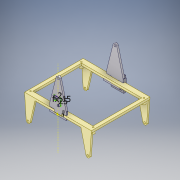
# Autodesk Inventor part: ControllerPCBHolder
Saved by Autodesk Inventor 2019.1 (Build 231200000, 200)
## iProperties
Created: 2018-09-15
Part Number: ControllerPCBHolder
Material: Generisch
Document SubType Name: Modeling
Designer: JochenAlt
Density: 1 g/cm^3
Appearance: Nylon 6
Author: JochenAlt
Autodesk Inventor part; units mm, degrees
ref_plane "YZ Plane" through (0, 0, 0) normal (1, 0, 0) x (0, 1, 0)
ref_plane "XZ Plane" through (0, 0, 0) normal (0, 1, 0) x (-1, 0, 0)
ref_plane "XY Plane" through (0, 0, 0) normal (0, 0, 1) x (1, 0, 0)
sketch "Skizze1" plane through (0, 0, 0) normal (0, 0, 1) x (1, 0, 0)
  line L0 (-61, 50.5) -> (61, 50.5)
  line L1 (61, 50.5) -> (61, -50.5)
  line L2 (61, -50.5) -> (-61, -50.5)
  line L3 (-61, -50.5) -> (-61, 50.5)
  line L4 (0, 70.7) -> (0, -70.7) construction
  line L5 (-85.4, 0) -> (85.4, 0) construction
  line L6 (-55, 44.5) -> (55, 44.5)
  line L7 (55, 44.5) -> (55, -44.5)
  line L8 (55, -44.5) -> (-55, -44.5)
  line L9 (-55, -44.5) -> (-55, 44.5)
  line L10 (-57.15, 46.36) -> (57.15, 46.36) construction
  line L11 (57.15, 46.36) -> (57.15, -46.36) construction
  line L12 (57.15, -46.36) -> (-57.15, -46.36) construction
  line L13 (-57.15, -46.36) -> (-57.15, 46.36) construction
  circle A0 centre (-57.15, 46.36) radius 1.25
  circle A1 centre (57.15, 46.36) radius 1.25
  circle A2 centre (-57.15, -46.36) radius 1.25
  circle A3 centre (57.15, -46.36) radius 1.25
  circle A4 centre (57.15, 46.36) radius 2.8429
  circle A5 centre (-57.15, 46.36) radius 2.8429
  circle A6 centre (-57.15, -46.36) radius 2.8429
  circle A7 centre (57.15, -46.36) radius 2.8429
  point P0 (0, 0)
  dimension "d0" = 122
  dimension "d1" = 101
  dimension "d4" = 6
  dimension "d5" = 6
  dimension "d6" = 2.5
  dimension "d7" = 114.3
  dimension "d8" = 92.72
  constraints: 24 end point, 8 coincident, 6 parallel, 4 centre point, 3 equal radius, 3 horizontal, 3 perpendicular, 18 other
  measures "d0" distance of L0.start L0.end
  measures "d1" distance of L0.end L1.end
  measures "d4" distance between parallel lines of L6 L0
  measures "d5" distance between parallel lines of L9 L3
  measures "d6" diameter of A0
  measures "d7" distance of L11.end L12.end
  measures "d8" distance of L10.end L11.end
extrude "Extrusion2" add sketch "Skizze1" along normal blind 4 contours L0 L1 L2 L3 | A4 | A7 | A6 | A5
extrude "Extrusion15" add sketch "Skizze1" against normal blind 5 contours A4 | A7 | A6 | A5
sketch "Skizze2" plane through (0, 0, 0) normal (0, 1, 0) x (-1, 0, 0)
  arc A0 (51.152, -39.299) -> (58.0513, -38.7409) centre (54.5596, -38.5) ccw
  arc A1 (-58.0513, -38.7409) -> (-51.152, -39.299) centre (-54.5596, -38.5) ccw
  line L0 (0, -100.1) -> (0, 86.1) construction
  line L1 (-93.1, 0) -> (93.1, 0) construction
  circle A2 centre (54.5596, -38.5) radius 1.75
  circle A3 centre (-54.5596, -38.5) radius 1.75
  line L2 (58.0513, -38.7409) -> (61, 4)
  line L3 (-58.0513, -38.7409) -> (-61, 4)
  line L4 (-61, 4) -> (61, 4) construction
  line L5 (61, 4) -> (41, 4)
  line L6 (-61, 4) -> (-41, 4)
  circle A4 centre (0, 56) radius 1.75
  arc A5 (3.3952, 56.8501) -> (-3.3952, 56.8501) centre (0, 56) ccw
  line L7 (54.5596, -38.5) -> (0, 56) construction
  line L8 (61, 0) -> (-61, 0) construction
  circle A6 centre (0, -7) radius 63 construction
  line L9 (54.5596, -38.5) -> (-54.5596, -38.5) construction
  line L10 (0, 56) -> (-54.5596, -38.5) construction
  line L11 (55, 4) -> (-55, 4) construction
  line L12 (7, 0) -> (7, 0)
  line L13 (7, 0) -> (-7, 0)
  line L14 (7, 4.5) -> (15, 4.5)
  line L15 (15, 4.5) -> (15, 10.0685)
  line L16 (-15, 10.0685) -> (-15, 4.5)
  line L17 (-15, 4.5) -> (-7, 4.5)
  line L18 (7, 9.5) -> (-7, 9.5)
  line L19 (7, 9.5) -> (7, 0)
  line L20 (-7, 9.5) -> (-7, 0)
  line L21 (-3.3952, 56.8501) -> (-14.8952, 10.9186)
  line L22 (3.3952, 56.8501) -> (14.8952, 10.9186)
  arc A7 (-14.8952, 10.9186) -> (-15, 10.0685) centre (-11.5, 10.0685) ccw
  arc A8 (15, 10.0685) -> (14.8952, 10.9186) centre (11.5, 10.0685) ccw
  line L23 (-51.152, -39.299) -> (-41, 4)
  line L24 (51.152, -39.299) -> (41, 4)
  line L25 (-61, 0) -> (-61, 4) projected
  circle A9 centre (0, -7) radius 66.5 construction
  point P0 (0, 0)
  point P1 (15, 10.5)
  dimension "d12" = 3.5
  dimension "d22" = 63
  dimension "d23" = 3.5
  dimension "d54" = 6
  dimension "d61" = 30
  dimension "d71" = 0.5
  dimension "d74" = 7
  dimension "d76" = 5
  dimension "d81" = 20
  dimension "d82" = 14
  dimension "d98" = 66.5
  constraints: 40 end point, 12 point on circle, 12 tangent, 10 centre point, 8 point on line, 6 equal radius, 5 horizontal, 5 midpoint, 3 coincident, 3 collinear, 2 equal length, 2 perpendicular, 1 vertical, 5 other
  measures "d12" diameter of A2
  measures "d22" radius of A6
  measures "d23" radius of A0
  measures "d54" distance of point (15, 10.5) L14.end
  measures "d61" distance between parallel lines of L16 L15
  measures "d71" distance between parallel lines of L11 L14
  measures "d74" distance from line of A6.centre L1
  measures "d76" distance between parallel lines of L18 L17
  measures "d81" distance of L6.end L3.end
  measures "d82" distance of L18.start L18.end
  measures "d98" radius of A9
extrude "Extrusion3" add sketch "Skizze2" along normal blind 3 from surface at 50.5 contours L24 L5 L2 A0 | L3 L6 L23 A1
extrude "Extrusion4" add sketch "Skizze2" against normal blind 3 from surface at -50.5 contours L24 L5 L2 A0 | L3 L6 L23 A1
sketch "Skizze4" plane through (0, 0, 0) normal (0, 0, 1) x (1, 0, 0)
  line L0 (-61, 53.5) -> (-61, 50.5) projected
  line L1 (41, -53.5) -> (61, -53.5) projected
  line L2 (-61, 53.5) -> (61, 53.5)
  line L3 (61, 53.5) -> (61, -53.5)
  line L4 (61, -53.5) -> (-61, -53.5)
  line L5 (-61, -53.5) -> (-61, 53.5)
  line L6 (61, -50.5) -> (61, 50.5) projected
  line L7 (61, -50.5) -> (-61, -50.5)
  line L8 (-61, -50.5) -> (-61, 50.5)
  line L9 (-61, 50.5) -> (61, 50.5)
  line L10 (61, 50.5) -> (61, -50.5)
  point P0 (0, 0)
  point P1 (-60.5133, 50.5)
  point P2 (55.6888, -53.5)
  constraints: 16 end point, 4 parallel, 2 horizontal, 2 perpendicular, 1 coincident, 1 other
extrude "Extrusion5" add sketch "Skizze4" along normal blind 4 contours L2 L3 L9 L0 | L7 L3 L1 L4 L5
extrude "Extrusion7" cut sketch "Skizze2" along normal up to surface (3 mm away) from surface at -53.5 contours A4 | L19 L13 L20 L18
extrude "Extrusion8" cut sketch "Skizze2" against normal up to surface (3 mm away) from surface at 53.5 contours A4 | L19 L13 L20 L18
sketch "Skizze5" plane through (0, 0, 0) normal (0, 1, 0) x (-1, 0, 0)
  point P0 (0, 0)
extrude "Extrusion6" add sketch "Skizze2" against normal up to surface (3 mm away) from surface at -50.5 separate body contours L22 A8 L15 L14 L19 L18 L20 L17 L16 A7 L21 A5 | L19 L13 L20 L18
extrude "Extrusion9" add sketch "Skizze2" against normal up to surface (3 mm away) from surface at 53.5 contours L22 A8 L15 L14 L19 L18 L20 L17 L16 A7 L21 A5 | L19 L13 L20 L18 bodies 2
sketch "Skizze7" plane through (4, -53.5, 0) normal (0, 0, -1) x (-1, 0, 0)
  line L0 (-37.9379, 0) -> (-3, 0) construction
  line L1 (19, 0) -> (19, 0)
  line L2 (-11, 0) -> (-11, 9)
  line L3 (-11, 9) -> (19, 9)
  line L4 (19, 9) -> (19, 0)
  line L5 (59, 9) -> (-51, 9) construction
  line L6 (19, 107) -> (-11, 107)
  line L7 (-11, 107) -> (-11, 98)
  line L8 (-11, 98) -> (19, 98)
  line L9 (19, 98) -> (19, 107)
  line L10 (59, 98) -> (-51, 98) projected
  line L11 (7.3952, 3) -> (7.3952, 0) construction
  line L12 (-0.5, 3) -> (-0.5, 0) construction
  line L13 (2.25, 3) -> (5.75, 3) construction
  line L14 (2.25, 0) -> (5.75, 0) construction
  line L15 (11, 3) -> (-3, 3) construction
  line L16 (4, 3) -> (4, 0) construction
  line L17 (7.3952, 0) -> (0.6048, 0) construction
  line L18 (19, 9) -> (19, 0)
  line L19 (19, 9) -> (19, 9)
  line L20 (19, 0) -> (-11, 0)
  point P0 (4, 53.5)
  point P1 (11.5, 0)
  point P2 (59.6888, 0)
  point P3 (-3.5, 107)
  point P4 (8.5, 3)
  point P5 (8.5, 0)
  point P6 (11.5, 3)
  point P7 (-51.6888, 0)
  point P8 (11, 3)
  dimension "d45" = 30
  dimension "d51" = 15
  constraints: 24 end point, 7 parallel, 3 horizontal, 3 perpendicular, 2 collinear, 2 point on line, 1 midpoint, 6 other
  measures "d45" distance between parallel lines of L2 L4
  measures "d51" distance between parallel lines of L16 L2
extrude "Extrusion10" add sketch "Skizze7" along normal blind 3 contours L9 L8 L7 L6 bodies 2
extrude "Extrusion12" add sketch "Skizze7" along normal blind 3 contours L2 L3 L4 L20 bodies 2
sketch "Skizze10" plane through (0, 53.5, 56) normal (0, 1, 0) x (1, 0, 0)
  line L0 (15, 59) -> (-15, 59)
  line L1 (-15, 59) -> (-15, 46.5)
  line L2 (-15, 46.5) -> (15, 46.5)
  line L3 (15, 46.5) -> (15, 59)
  line L4 (14.8952, 45.0814) -> (3.3952, -0.8501) projected
  line L5 (-3.3952, -0.8501) -> (-14.8952, 45.0814) projected
  point P0 (0, 56)
  point P1 (-15, 45.9315)
  constraints: 8 end point, 3 perpendicular, 1 coincident, 1 horizontal
extrude "Extrusion14" add sketch "Skizze10" along normal blind 3 bodies 2
sketch "Skizze6" plane through (-55.6888, 56.5, -8.5) normal (0, -1, 0) x (1, 0, 0)
  line L0 (-29.7112, 8.5) -> (141.0888, 8.5) construction
  line L1 (55.6888, 88.3) -> (55.6888, -53.8) construction
  line L2 (44.6888, 9) -> (63.6888, 9)
  line L3 (63.6888, 9) -> (63.6888, -7)
  line L4 (63.6888, -7) -> (44.6888, -7)
  line L5 (44.6888, -7) -> (44.6888, 9)
  circle A0 centre (47.1888, -4.5) radius 1.75
  circle A1 centre (61.1888, -4.5) radius 1.75
  line L6 (61.1888, -4.5) -> (47.1888, -4.5) construction
  line L7 (54.1888, 9) -> (54.1888, -7) construction
  line L8 (42.6888, -9) -> (65.6888, -9)
  line L9 (65.6888, -9) -> (65.6888, 11)
  line L10 (65.6888, 11) -> (42.6888, 11)
  line L11 (42.6888, 11) -> (42.6888, -9)
  circle A2 centre (61.1888, -4.5) radius 3.25
  circle A3 centre (47.1888, -4.5) radius 3.25
  line L12 (42.6888, 11) -> (42.6888, 18)
  line L13 (42.6888, 18) -> (65.6888, 18)
  line L14 (65.6888, 18) -> (65.6888, 11)
  line L15 (40.6888, 18) -> (70.6888, 18) projected
  point P0 (55.6888, 1.5)
  point P1 (40.6888, 14.5)
  point P2 (70.6888, 14.088)
  point P3 (40.6888, 14.5)
  point P4 (70.6888, 14.5)
  dimension "d24" = 19
  dimension "d25" = 16
  dimension "d30" = 3.5
  dimension "d31" = 2.5
  dimension "d32" = 14
  dimension "d33" = 8
  dimension "d48" = 2
  dimension "d58" = 1.5
  dimension "d69" = 7.5
  constraints: 26 end point, 5 perpendicular, 4 centre point, 4 parallel, 2 coincident, 2 equal radius, 2 horizontal, 2 midpoint, 1 symmetric about line, 1 vertical, 6 other
  measures "d24" distance of L3.end L4.end
  measures "d25" distance of L2.end L3.end
  measures "d30" diameter of A0
  measures "d31" distance from line of L4 L6.start
  measures "d32" distance of L6.start L6.end
  measures "d33" distance between parallel lines of L3 L1
  measures "d48" distance between parallel lines of L4 L8
  measures "d58" radial gap between concentric circles of A2 A1
  measures "d69" distance from line of L2 point (55.689, 1.5)
extrude "Extrusion11" add sketch "Skizze6" against normal blind 4 contours L2 L3 A2 L4 A3 L5 | A3 L4 L5 | L5 A3 | A2 L3 | L3 A2 L4 | A3 L4 L5 | L3 L4 A2 | L4 A2 | L4 A3 | L11 L10 L9 L8 | L12 L13 L14 L10 bodies 2
extrude "Extrusion13" add sketch "Skizze6" against normal blind 4 from surface at -4 contours A3 L4 L5 | L5 A3 | A2 L3 | L3 A2 L4 | L4 A2 | L4 A3 picked at (47.2591, -6.7457) picked at (61.1185, -6.7457) bodies 2
sketch "Skizze11" plane through (0, -53.5, 56) normal (0, 1, 0) x (1, 0, 0)
  line L0 (2.7849, 27.4336) -> (2.7849, 29)
  line L1 (3.7849, 33.143) -> (3.7849, 42.4336) construction
  line L2 (-7.2367, 35.2067) -> (-1.2709, 35.2067) construction
  line L3 (-1.2709, 35.2067) -> (-1.2709, 30.6706) construction
  line L4 (-1.2709, 30.6706) -> (-7.2367, 30.6706) construction
  line L5 (-7.2367, 30.6706) -> (-7.2367, 35.2067) construction
  line L6 (-5.7414, 31) -> (2.7849, 31)
  line L7 (6.3513, 31) -> (6.3513, 29)
  line L8 (-5.7414, 29) -> (-5.7414, 28)
  line L9 (-5.7414, 28) -> (-8.6487, 30)
  line L10 (-8.6487, 30) -> (-5.7414, 32)
  line L11 (-5.7414, 32) -> (-5.7414, 31)
  line L12 (-8.6487, 30) -> (6.3513, 30) construction
  line L13 (-0.9289, 43.4415) -> (1.8143, 43.4415) construction
  line L14 (1.8143, 43.4415) -> (1.8143, 38.6749) construction
  line L15 (1.8143, 38.6749) -> (-0.9289, 38.6749) construction
  line L16 (-0.9289, 38.6749) -> (-0.9289, 43.4415) construction
  line L17 (2.7849, 31) -> (2.7849, 39.5263)
  line L18 (4.7849, 31) -> (6.3513, 31)
  line L19 (4.7849, 39.5263) -> (4.7849, 31)
  line L20 (4.7849, 29) -> (4.7849, 27.4336)
  line L21 (6.3513, 29) -> (4.7849, 29)
  line L22 (-7.1951, 29) -> (-5.7414, 29) construction
  line L23 (0, 118.3) -> (0, -23.8) construction
  line L24 (4.7849, 39.5263) -> (5.7849, 39.5263)
  line L25 (5.7849, 39.5263) -> (3.7849, 42.4336)
  line L26 (3.7849, 42.4336) -> (1.7849, 39.5263)
  line L27 (1.7849, 39.5263) -> (2.7849, 39.5263)
  line L28 (4.7849, 27.4336) -> (2.7849, 27.4336)
  line L29 (-7, 56) -> (7, 56) projected
  line L30 (2.7849, 29) -> (-5.7414, 29)
  line L31 (-3.9125, 31.7067) -> (-4.9279, 31.7067)
  line L32 (-4.9279, 31.7067) -> (-5.603, 32.8214)
  line L33 (-5.603, 32.8214) -> (-6.2922, 31.7067)
  line L34 (-6.2922, 31.7067) -> (-7.265, 31.7067)
  line L35 (-7.265, 31.7067) -> (-6.1277, 33.4681)
  line L36 (-6.1277, 33.4681) -> (-7.2197, 35.2067)
  line L37 (-7.2197, 35.2067) -> (-6.2043, 35.2067)
  line L38 (-6.2043, 35.2067) -> (-5.5718, 34.1488)
  line L39 (-5.5718, 34.1488) -> (-4.9223, 35.2067)
  line L40 (-4.9223, 35.2067) -> (-3.9494, 35.2067)
  line L41 (-3.9494, 35.2067) -> (-5.047, 33.505)
  line L42 (-5.047, 33.505) -> (-3.9125, 31.7067)
  line L43 (2.3442, 43.4415) -> (1.1359, 41.4022)
  line L44 (1.1359, 41.4022) -> (1.1359, 39.9415)
  line L45 (1.1359, 39.9415) -> (0.2567, 39.9415)
  line L46 (0.2567, 39.9415) -> (0.2567, 41.3597)
  line L47 (0.2567, 41.3597) -> (-0.9714, 43.4415)
  line L48 (-0.9714, 43.4415) -> (0.0298, 43.4415)
  line L49 (0.0298, 43.4415) -> (0.7133, 42.1936)
  line L50 (0.7133, 42.1936) -> (1.3742, 43.4415)
  line L51 (1.3742, 43.4415) -> (2.3442, 43.4415)
  point P0 (0, 56)
  point P1 (-4.2538, 35.2067)
  dimension "d92" = 25
  dimension "d93" = 2
  dimension "d95" = 15
  constraints: 42 end point, 7 parallel, 6 equal length, 5 collinear, 5 perpendicular, 3 horizontal, 3 midpoint, 2 point on line, 1 vertical, 7 other
  measures "d92" distance between parallel lines of L18 L29
  measures "d93" distance of L20.end L0.start
  measures "d95" distance from line of L28 L1.end
extrude "Extrusion16" add sketch "Skizze11" against normal blind 1 bodies 2
equation "\"d5\" = d4"
